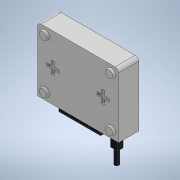
# Autodesk Inventor part: RB941-2nD
Saved by Autodesk Inventor 2022 (Build 260153000, 153)
## iProperties
Created: 2017-05-26
Part Number: RB941-2nD
Material: Ogólne
Document SubType Name: Modeling
Designer: SewerLight
Density: 1 g/cm^3
Appearance: Domyślne
Author: SewerLight
Autodesk Inventor part; units mm, degrees
ref_plane "XZ Plane" through (0, 0, 0) normal (0, 1, 0) x (-1, 0, 0)
sketch "Szkic1" plane through (0, 0, 0) normal (0, 1, 0) x (-1, 0, 0)
  line L0 (56.5, -44.5) -> (-56.5, -44.5)
  line L1 (-56.5, -44.5) -> (-56.5, 44.5)
  line L2 (-56.5, 44.5) -> (56.5, 44.5)
  line L3 (56.5, 44.5) -> (56.5, -44.5)
  line L4 (56.5, -44.5) -> (-56.5, 44.5) construction
  line L5 (-56.5, -44.5) -> (56.5, 44.5) construction
  point P0 (0, 0)
  dimension "d0" = 113
  dimension "d1" = 89
  constraints: 12 end point, 2 midpoint, 2 parallel, 1 horizontal, 1 perpendicular
  measures "d0" distance of L1.end L2.end
  measures "d1" distance of L0.end L1.end
extrude "Wyciągnięcie proste1" add sketch "Szkic1" along normal blind 28
sketch "Szkic2" plane through (0, 28, 0) normal (0, 1, 0) x (1, 0, 0)
  line L0 (56.5, 44.5) -> (56.5, -44.5) projected
  line L1 (56.5, -44.5) -> (-56.5, -44.5) projected
  line L2 (-56.5, -44.5) -> (-56.5, 44.5) projected
  line L3 (-56.5, 44.5) -> (56.5, 44.5) projected
  line L4 (-56.5, 44.5) -> (56.5, 44.5) construction
  line L5 (56.5, 44.5) -> (56.5, -44.5) construction
  line L6 (56.5, -44.5) -> (-56.5, -44.5) construction
  line L7 (-56.5, -44.5) -> (-56.5, 44.5) construction
  line L8 (-25.5673, 3.2324) -> (-27.2934, 3.2324)
  line L9 (-27.2934, 3.2324) -> (-30.4538, 7.2113)
  line L10 (-30.4538, 7.2113) -> (-31.9773, 7.2113)
  line L11 (-31.9773, 7.2113) -> (-31.9773, 3.2324)
  line L12 (-31.9773, 3.2324) -> (-33.3063, 3.2324)
  line L13 (-33.3063, 3.2324) -> (-33.3063, 13.2324)
  line L14 (-33.3063, 13.2324) -> (-30.7293, 13.2324)
  spline S0 degree 2 poles (-30.7293, 13.2324) (-29.8703, 13.2324) (-28.7115, 13.046) (-28.1848, 12.7056) knots 0 0 0 1 2 2 2
  spline S1 degree 2 poles (-28.1848, 12.7056) (-27.658, 12.3653) (-27.0502, 11.3037) (-27.0502, 10.5176) knots 0 0 0 1 2 2 2
  spline S2 degree 2 poles (-27.0502, 10.5176) (-27.0502, 9.4236) (-28.1686, 7.9406) (-29.1248, 7.5841) knots 0 0 0 1 2 2 2
  line L15 (-29.1248, 7.5841) -> (-25.5673, 3.2324)
  spline S3 degree 2 poles (-28.436, 10.4123) (-28.436, 10.8499) (-28.7439, 11.5225) (-29.0681, 11.7413) knots 0 0 0 1 2 2 2
  spline S4 degree 2 poles (-29.0681, 11.7413) (-29.3517, 11.9277) (-30.1053, 12.0816) (-30.6564, 12.0816) knots 0 0 0 1 2 2 2
  line L16 (-30.6564, 12.0816) -> (-31.9773, 12.0816)
  line L17 (-31.9773, 12.0816) -> (-31.9773, 8.3215)
  line L18 (-31.9773, 8.3215) -> (-30.8104, 8.3215)
  spline S5 degree 2 poles (-30.8104, 8.3215) (-30.235, 8.3215) (-29.3193, 8.5241) (-29.0032, 8.8401) knots 0 0 0 1 2 2 2
  spline S6 degree 2 poles (-29.0032, 8.8401) (-28.7115, 9.1157) (-28.436, 9.8936) (-28.436, 10.4123) knots 0 0 0 1 2 2 2
  spline S7 degree 2 poles (-17.9903, 6.3037) (-17.9903, 5.5581) (-18.5575, 4.4155) (-19.0276, 4.0427) knots 0 0 0 1 2 2 2
  spline S8 degree 2 poles (-19.0276, 4.0427) (-19.5948, 3.6051) (-20.8833, 3.2324) (-21.9044, 3.2324) knots 0 0 0 1 2 2 2
  line L19 (-21.9044, 3.2324) -> (-24.7731, 3.2324)
  line L20 (-24.7731, 3.2324) -> (-24.7731, 13.2324)
  line L21 (-24.7731, 13.2324) -> (-22.1232, 13.2324)
  spline S9 degree 2 poles (-22.1232, 13.2324) (-21.0535, 13.2324) (-19.9838, 13.0946) (-19.4976, 12.8272) knots 0 0 0 1 2 2 2
  spline S10 degree 2 poles (-19.4976, 12.8272) (-18.9546, 12.5436) (-18.4603, 11.6116) (-18.4603, 10.9795) knots 0 0 0 1 2 2 2
  spline S11 degree 2 poles (-18.4603, 10.9795) (-18.4603, 10.2745) (-19.2058, 9.1562) (-19.8622, 8.8401) knots 0 0 0 1 2 2 2
  line L22 (-19.8622, 8.8401) -> (-19.8622, 8.7915)
  spline S12 degree 2 poles (-19.8622, 8.7915) (-18.9708, 8.5484) (-17.9903, 7.2599) (-17.9903, 6.3037) knots 0 0 0 1 2 2 2
  spline S13 degree 2 poles (-19.376, 6.247) (-19.376, 6.8142) (-19.7002, 7.5436) (-20.1864, 7.8029) knots 0 0 0 1 2 2 2
  spline S14 degree 2 poles (-20.1864, 7.8029) (-20.5024, 7.9649) (-21.248, 8.0622) (-21.9368, 8.0622) knots 0 0 0 1 2 2 2
  line L23 (-21.9368, 8.0622) -> (-23.4441, 8.0622)
  line L24 (-23.4441, 8.0622) -> (-23.4441, 4.3669)
  line L25 (-23.4441, 4.3669) -> (-22.3663, 4.3669)
  spline S15 degree 2 poles (-22.3663, 4.3669) (-21.4911, 4.3669) (-20.4862, 4.529) (-20.0972, 4.7883) knots 0 0 0 1 2 2 2
  spline S16 degree 2 poles (-20.0972, 4.7883) (-19.7245, 5.0557) (-19.376, 5.7202) (-19.376, 6.247) knots 0 0 0 1 2 2 2
  spline S17 degree 2 poles (-19.846, 10.7931) (-19.846, 11.1497) (-20.0891, 11.6846) (-20.3566, 11.8385) knots 0 0 0 1 2 2 2
  spline S18 degree 2 poles (-20.3566, 11.8385) (-20.6807, 12.0168) (-21.4668, 12.0978) (-22.1718, 12.0978) knots 0 0 0 1 2 2 2
  line L26 (-22.1718, 12.0978) -> (-23.4441, 12.0978)
  line L27 (-23.4441, 12.0978) -> (-23.4441, 9.1724)
  line L28 (-23.4441, 9.1724) -> (-21.9368, 9.1724)
  spline S19 degree 2 poles (-21.9368, 9.1724) (-21.3128, 9.1724) (-20.7212, 9.3021) (-20.4052, 9.5047) knots 0 0 0 1 2 2 2
  spline S20 degree 2 poles (-20.4052, 9.5047) (-20.0972, 9.6991) (-19.846, 10.3231) (-19.846, 10.7931) knots 0 0 0 1 2 2 2
  spline S21 degree 2 poles (-17.2285, 9.9828) (-17.2285, 10.7526) (-16.7261, 12.033) (-16.2885, 12.4949) knots 0 0 0 1 2 2 2
  spline S22 degree 2 poles (-16.2885, 12.4949) (-15.8752, 12.9406) (-14.6677, 13.435) (-14.0519, 13.435) knots 0 0 0 1 2 2 2
  spline S23 degree 2 poles (-14.0519, 13.435) (-13.363, 13.435) (-12.2447, 12.973) (-11.8314, 12.5354) knots 0 0 0 1 2 2 2
  spline S24 degree 2 poles (-11.8314, 12.5354) (-11.3128, 11.9844) (-10.7455, 10.2016) (-10.7455, 8.832) knots 0 0 0 1 2 2 2
  spline S25 degree 2 poles (-10.7455, 8.832) (-10.7455, 7.5922) (-11.3047, 5.3718) (-11.8476, 4.6343) knots 0 0 0 1 2 2 2
  spline S26 degree 2 poles (-11.8476, 4.6343) (-12.423, 3.8564) (-14.0438, 3.0379) (-15.2269, 3.0379) knots 0 0 0 1 2 2 2
  spline S27 degree 2 poles (-15.2269, 3.0379) (-15.4943, 3.0379) (-16.1021, 3.0946) (-16.3614, 3.1756) knots 0 0 0 1 2 2 2
  line L29 (-16.3614, 3.1756) -> (-16.3614, 4.4641)
  line L30 (-16.3614, 4.4641) -> (-16.2966, 4.4641)
  spline S28 degree 2 poles (-16.2966, 4.4641) (-16.1264, 4.3669) (-15.4133, 4.1967) (-15.0486, 4.1967) knots 0 0 0 1 2 2 2
  spline S29 degree 2 poles (-15.0486, 4.1967) (-13.7358, 4.1967) (-12.2366, 5.9309) (-12.1313, 7.5354) knots 0 0 0 1 2 2 2
  spline S30 degree 2 poles (-12.1313, 7.5354) (-12.6661, 7.1708) (-13.6386, 6.8385) (-14.2139, 6.8385) knots 0 0 0 1 2 2 2
  spline S31 degree 2 poles (-14.2139, 6.8385) (-14.765, 6.8385) (-15.6807, 7.0816) (-16.1426, 7.4301) knots 0 0 0 1 2 2 2
  spline S32 degree 2 poles (-16.1426, 7.4301) (-16.6775, 7.8434) (-17.2285, 9.0995) (-17.2285, 9.9828) knots 0 0 0 1 2 2 2
  spline S33 degree 2 poles (-12.0989, 9.1319) (-12.0989, 10.1448) (-12.4716, 11.4252) (-12.8039, 11.7737) knots 0 0 0 1 2 2 2
  spline S34 degree 2 poles (-12.8039, 11.7737) (-13.0956, 12.0978) (-13.7034, 12.341) (-14.06, 12.341) knots 0 0 0 1 2 2 2
  spline S35 degree 2 poles (-14.06, 12.341) (-14.8865, 12.341) (-15.8671, 11.1578) (-15.8671, 10.0395) knots 0 0 0 1 2 2 2
  spline S36 degree 2 poles (-15.8671, 10.0395) (-15.8671, 9.4074) (-15.5429, 8.5889) (-15.1864, 8.2972) knots 0 0 0 1 2 2 2
  spline S37 degree 2 poles (-15.1864, 8.2972) (-14.9271, 8.0865) (-14.2869, 7.9487) (-13.9141, 7.9487) knots 0 0 0 1 2 2 2
  spline S38 degree 2 poles (-13.9141, 7.9487) (-13.4846, 7.9487) (-12.4959, 8.2486) (-12.1232, 8.4998) knots 0 0 0 1 2 2 2
  spline S39 degree 2 poles (-12.1232, 8.4998) (-12.1151, 8.597) (-12.0989, 8.9293) (-12.0989, 9.1319) knots 0 0 0 1 2 2 2
  line L31 (-3.0146, 6.6683) -> (-4.2058, 6.6683)
  line L32 (-4.2058, 6.6683) -> (-4.2058, 3.2324)
  line L33 (-4.2058, 3.2324) -> (-5.4943, 3.2324)
  line L34 (-5.4943, 3.2324) -> (-5.4943, 6.6683)
  line L35 (-5.4943, 6.6683) -> (-9.9109, 6.6683)
  line L36 (-9.9109, 6.6683) -> (-9.9109, 8.0784)
  line L37 (-9.9109, 8.0784) -> (-5.4376, 13.2324)
  line L38 (-5.4376, 13.2324) -> (-4.2058, 13.2324)
  line L39 (-4.2058, 13.2324) -> (-4.2058, 7.7461)
  line L40 (-4.2058, 7.7461) -> (-3.0146, 7.7461)
  line L41 (-3.0146, 7.7461) -> (-3.0146, 6.6683)
  line L42 (-5.4943, 7.7461) -> (-5.4943, 11.6521)
  line L43 (-5.4943, 11.6521) -> (-8.8574, 7.7461)
  line L44 (-8.8574, 7.7461) -> (-5.4943, 7.7461)
  line L45 (3.7196, 3.2324) -> (-1.1588, 3.2324)
  line L46 (-1.1588, 3.2324) -> (-1.1588, 4.2534)
  line L47 (-1.1588, 4.2534) -> (0.6564, 4.2534)
  line L48 (0.6564, 4.2534) -> (0.6564, 10.9552)
  line L49 (0.6564, 10.9552) -> (-1.1588, 10.9552)
  line L50 (-1.1588, 10.9552) -> (-1.1588, 11.8709)
  spline S40 degree 2 poles (-1.1588, 11.8709) (-0.1297, 11.8709) (0.8428, 12.4544) (0.9076, 13.2648) knots 0 0 0 1 2 2 2
  line L51 (0.9076, 13.2648) -> (1.9449, 13.2648)
  line L52 (1.9449, 13.2648) -> (1.9449, 4.2534)
  line L53 (1.9449, 4.2534) -> (3.7196, 4.2534)
  line L54 (3.7196, 4.2534) -> (3.7196, 3.2324)
  line L55 (9.222, 7.0006) -> (5.4376, 7.0006)
  line L56 (5.4376, 7.0006) -> (5.4376, 8.2162)
  line L57 (5.4376, 8.2162) -> (9.222, 8.2162)
  line L58 (9.222, 8.2162) -> (9.222, 7.0006)
  line L59 (16.718, 3.2324) -> (10.5511, 3.2324)
  line L60 (10.5511, 3.2324) -> (10.5511, 4.6505)
  spline S41 degree 2 poles (10.5511, 4.6505) (11.2156, 5.2745) (12.3987, 6.4333) (12.966, 7.0573) knots 0 0 0 1 2 2 2
  spline S42 degree 2 poles (12.966, 7.0573) (14.1086, 8.3134) (14.9433, 9.8207) (14.9433, 10.623) knots 0 0 0 1 2 2 2
  spline S43 degree 2 poles (14.9433, 10.623) (14.9433, 11.0444) (14.684, 11.6765) (14.4489, 11.879) knots 0 0 0 1 2 2 2
  spline S44 degree 2 poles (14.4489, 11.879) (14.2139, 12.0816) (13.5981, 12.2842) (13.2253, 12.2842) knots 0 0 0 1 2 2 2
  spline S45 degree 2 poles (13.2253, 12.2842) (12.8687, 12.2842) (12.1394, 12.106) (11.8071, 11.9682) knots 0 0 0 1 2 2 2
  spline S46 degree 2 poles (11.8071, 11.9682) (11.5235, 11.8547) (10.9968, 11.5306) (10.8347, 11.4171) knots 0 0 0 1 2 2 2
  line L61 (10.8347, 11.4171) -> (10.7618, 11.4171)
  line L62 (10.7618, 11.4171) -> (10.7618, 12.8434)
  spline S47 degree 2 poles (10.7618, 12.8434) (11.175, 13.046) (12.658, 13.4431) (13.3225, 13.4431) knots 0 0 0 1 2 2 2
  spline S48 degree 2 poles (13.3225, 13.4431) (14.7245, 13.4431) (16.3047, 11.9601) (16.3047, 10.6959) knots 0 0 0 1 2 2 2
  spline S49 degree 2 poles (16.3047, 10.6959) (16.3047, 10.1043) (16.0292, 9.1157) (15.7861, 8.6943) knots 0 0 0 1 2 2 2
  spline S50 degree 2 poles (15.7861, 8.6943) (15.543, 8.2567) (14.8379, 7.3977) (14.4489, 6.9844) knots 0 0 0 1 2 2 2
  spline S51 degree 2 poles (14.4489, 6.9844) (13.8169, 6.2956) (12.269, 4.8207) (11.8071, 4.3912) knots 0 0 0 1 2 2 2
  line L63 (11.8071, 4.3912) -> (16.718, 4.3912)
  line L64 (16.718, 4.3912) -> (16.718, 3.2324)
  line L65 (24.1329, 3.2324) -> (22.8687, 3.2324)
  line L66 (22.8687, 3.2324) -> (22.8687, 7.5111)
  spline S52 degree 2 poles (22.8687, 7.5111) (22.8687, 8.0298) (22.7715, 8.9212) (22.6256, 9.1886) knots 0 0 0 1 2 2 2
  spline S53 degree 2 poles (22.6256, 9.1886) (22.4716, 9.4722) (21.9206, 9.7478) (21.4506, 9.7478) knots 0 0 0 1 2 2 2
  spline S54 degree 2 poles (21.4506, 9.7478) (20.9806, 9.7478) (19.9838, 9.2453) (19.5057, 8.8401) knots 0 0 0 1 2 2 2
  line L67 (19.5057, 8.8401) -> (19.5057, 3.2324)
  line L68 (19.5057, 3.2324) -> (18.2415, 3.2324)
  line L69 (18.2415, 3.2324) -> (18.2415, 10.7364)
  line L70 (18.2415, 10.7364) -> (19.5057, 10.7364)
  line L71 (19.5057, 10.7364) -> (19.5057, 9.9017)
  spline S55 degree 2 poles (19.5057, 9.9017) (20.0729, 10.4123) (21.1669, 10.9471) (21.7828, 10.9471) knots 0 0 0 1 2 2 2
  spline S56 degree 2 poles (21.7828, 10.9471) (22.8849, 10.9471) (24.1329, 9.4884) (24.1329, 8.1027) knots 0 0 0 1 2 2 2
  line L72 (24.1329, 8.1027) -> (24.1329, 3.2324)
  spline S57 degree 2 poles (33.8898, 8.2243) (33.8898, 6.8547) (32.7796, 4.6505) (31.8477, 4.0346) knots 0 0 0 1 2 2 2
  spline S58 degree 2 poles (31.8477, 4.0346) (31.0859, 3.5565) (29.5219, 3.2324) (28.3063, 3.2324) knots 0 0 0 1 2 2 2
  line L73 (28.3063, 3.2324) -> (26.0049, 3.2324)
  line L74 (26.0049, 3.2324) -> (26.0049, 13.2324)
  line L75 (26.0049, 13.2324) -> (28.282, 13.2324)
  spline S59 degree 2 poles (28.282, 13.2324) (29.6921, 13.2324) (31.2966, 12.811) (31.8639, 12.4382) knots 0 0 0 1 2 2 2
  spline S60 degree 2 poles (31.8639, 12.4382) (32.8282, 11.798) (33.8898, 9.6829) (33.8898, 8.2243) knots 0 0 0 1 2 2 2
  spline S61 degree 2 poles (32.5041, 8.2405) (32.5041, 9.3912) (31.7423, 11.0201) (30.9887, 11.482) knots 0 0 0 1 2 2 2
  spline S62 degree 2 poles (30.9887, 11.482) (30.4538, 11.798) (29.2464, 12.0816) (28.3468, 12.0816) knots 0 0 0 1 2 2 2
  line L76 (28.3468, 12.0816) -> (27.3339, 12.0816)
  line L77 (27.3339, 12.0816) -> (27.3339, 4.3831)
  line L78 (27.3339, 4.3831) -> (28.3468, 4.3831)
  spline S63 degree 2 poles (28.3468, 4.3831) (29.2301, 4.3831) (30.5673, 4.6667) (31.1102, 5.0476) knots 0 0 0 1 2 2 2
  spline S64 degree 2 poles (31.1102, 5.0476) (31.8071, 5.5176) (32.5041, 7.0735) (32.5041, 8.2405) knots 0 0 0 1 2 2 2
  line L79 (-15.9319, -13.2324) -> (-17.2609, -13.2324)
  line L80 (-17.2609, -13.2324) -> (-17.2609, -4.6181)
  line L81 (-17.2609, -4.6181) -> (-19.8703, -10.4771)
  line L82 (-19.8703, -10.4771) -> (-20.6807, -10.4771)
  line L83 (-20.6807, -10.4771) -> (-23.2658, -4.6181)
  line L84 (-23.2658, -4.6181) -> (-23.2658, -13.2324)
  line L85 (-23.2658, -13.2324) -> (-24.5057, -13.2324)
  line L86 (-24.5057, -13.2324) -> (-24.5057, -3.2324)
  line L87 (-24.5057, -3.2324) -> (-22.6904, -3.2324)
  line L88 (-22.6904, -3.2324) -> (-20.1945, -8.7996)
  line L89 (-20.1945, -8.7996) -> (-17.7796, -3.2324)
  line L90 (-17.7796, -3.2324) -> (-15.9319, -3.2324)
  line L91 (-15.9319, -3.2324) -> (-15.9319, -13.2324)
  line L92 (-12.7147, -13.2324) -> (-13.9789, -13.2324)
  line L93 (-13.9789, -13.2324) -> (-13.9789, -5.7283)
  line L94 (-13.9789, -5.7283) -> (-12.7147, -5.7283)
  line L95 (-12.7147, -5.7283) -> (-12.7147, -13.2324)
  line L96 (-12.6256, -4.4803) -> (-14.06, -4.4803)
  line L97 (-14.06, -4.4803) -> (-14.06, -3.1675)
  line L98 (-14.06, -3.1675) -> (-12.6256, -3.1675)
  line L99 (-12.6256, -3.1675) -> (-12.6256, -4.4803)
  line L100 (-4.6434, -13.2324) -> (-6.3047, -13.2324)
  line L101 (-6.3047, -13.2324) -> (-9.0924, -9.61)
  line L102 (-9.0924, -9.61) -> (-9.5948, -10.0962)
  line L103 (-9.5948, -10.0962) -> (-9.5948, -13.2324)
  line L104 (-9.5948, -13.2324) -> (-10.859, -13.2324)
  line L105 (-10.859, -13.2324) -> (-10.859, -2.7867)
  line L106 (-10.859, -2.7867) -> (-9.5948, -2.7867)
  line L107 (-9.5948, -2.7867) -> (-9.5948, -8.8969)
  line L108 (-9.5948, -8.8969) -> (-6.6288, -5.7283)
  line L109 (-6.6288, -5.7283) -> (-5.0567, -5.7283)
  line L110 (-5.0567, -5.7283) -> (-8.1361, -8.8645)
  line L111 (-8.1361, -8.8645) -> (-4.6434, -13.2324)
  line L112 (-0.0324, -7.0816) -> (-0.0972, -7.0816)
  spline S65 degree 2 poles (-0.0972, -7.0816) (-0.2431, -7.0411) (-0.5592, -7.0249) (-0.778, -7.0249) knots 0 0 0 1 2 2 2
  spline S66 degree 2 poles (-0.778, -7.0249) (-1.2885, -7.0249) (-2.2934, -7.4706) (-2.7472, -7.9082) knots 0 0 0 1 2 2 2
  line L113 (-2.7472, -7.9082) -> (-2.7472, -13.2324)
  line L114 (-2.7472, -13.2324) -> (-4.0113, -13.2324)
  line L115 (-4.0113, -13.2324) -> (-4.0113, -5.7283)
  line L116 (-4.0113, -5.7283) -> (-2.7472, -5.7283)
  line L117 (-2.7472, -5.7283) -> (-2.7472, -6.8466)
  spline S67 degree 2 poles (-2.7472, -6.8466) (-2.0583, -6.2307) (-1.0292, -5.7283) (-0.543, -5.7283) knots 0 0 0 1 2 2 2
  spline S68 degree 2 poles (-0.543, -5.7283) (-0.3485, -5.7283) (-0.154, -5.7445) (-0.0324, -5.7688) knots 0 0 0 1 2 2 2
  line L118 (-0.0324, -5.7688) -> (-0.0324, -7.0816)
  spline S69 degree 2 poles (7.1151, -9.4803) (7.1151, -11.3766) (5.2917, -13.4431) (3.7682, -13.4431) knots 0 0 0 1 2 2 2
  spline S70 degree 2 poles (3.7682, -13.4431) (2.2042, -13.4431) (0.4133, -11.3118) (0.4133, -9.4803) knots 0 0 0 1 2 2 2
  spline S71 degree 2 poles (0.4133, -9.4803) (0.4133, -7.6003) (2.2609, -5.5176) (3.7682, -5.5176) knots 0 0 0 1 2 2 2
  spline S72 degree 2 poles (3.7682, -5.5176) (5.2917, -5.5176) (7.1151, -7.5922) (7.1151, -9.4803) knots 0 0 0 1 2 2 2
  spline S73 degree 2 poles (5.8104, -9.4803) (5.8104, -8.0217) (4.7488, -6.6035) (3.7682, -6.6035) knots 0 0 0 1 2 2 2
  spline S74 degree 2 poles (3.7682, -6.6035) (2.7877, -6.6035) (1.718, -8.0217) (1.718, -9.4803) knots 0 0 0 1 2 2 2
  spline S75 degree 2 poles (1.718, -9.4803) (1.718, -10.8985) (2.7877, -12.3572) (3.7682, -12.3572) knots 0 0 0 1 2 2 2
  spline S76 degree 2 poles (3.7682, -12.3572) (4.7407, -12.3572) (5.8104, -10.9228) (5.8104, -9.4803) knots 0 0 0 1 2 2 2
  line L119 (10.8428, -13.2324) -> (10.8428, -4.4155)
  line L120 (10.8428, -4.4155) -> (7.4878, -4.4155)
  line L121 (7.4878, -4.4155) -> (7.4878, -3.2324)
  line L122 (7.4878, -3.2324) -> (15.5267, -3.2324)
  line L123 (15.5267, -3.2324) -> (15.5267, -4.4155)
  line L124 (15.5267, -4.4155) -> (12.1718, -4.4155)
  line L125 (12.1718, -4.4155) -> (12.1718, -13.2324)
  line L126 (12.1718, -13.2324) -> (10.8428, -13.2324)
  line L127 (17.731, -13.2324) -> (16.4668, -13.2324)
  line L128 (16.4668, -13.2324) -> (16.4668, -5.7283)
  line L129 (16.4668, -5.7283) -> (17.731, -5.7283)
  line L130 (17.731, -5.7283) -> (17.731, -13.2324)
  line L131 (17.8201, -4.4803) -> (16.3857, -4.4803)
  line L132 (16.3857, -4.4803) -> (16.3857, -3.1675)
  line L133 (16.3857, -3.1675) -> (17.8201, -3.1675)
  line L134 (17.8201, -3.1675) -> (17.8201, -4.4803)
  line L135 (25.8023, -13.2324) -> (24.141, -13.2324)
  line L136 (24.141, -13.2324) -> (21.3533, -9.61)
  line L137 (21.3533, -9.61) -> (20.8509, -10.0962)
  line L138 (20.8509, -10.0962) -> (20.8509, -13.2324)
  line L139 (20.8509, -13.2324) -> (19.5867, -13.2324)
  line L140 (19.5867, -13.2324) -> (19.5867, -2.7867)
  line L141 (19.5867, -2.7867) -> (20.8509, -2.7867)
  line L142 (20.8509, -2.7867) -> (20.8509, -8.8969)
  line L143 (20.8509, -8.8969) -> (23.8169, -5.7283)
  line L144 (23.8169, -5.7283) -> (25.389, -5.7283)
  line L145 (25.389, -5.7283) -> (22.3096, -8.8645)
  line L146 (22.3096, -8.8645) -> (25.8023, -13.2324)
  point P0 (0, 0)
  constraints: 2 coincident, 2 other
emboss "Wypukłość1" sketch "Szkic2" operation add depth 0.1 direction (0, -1, 0) contours L8 L9 L10 L11 L12 L13 L14 S0 S1 S2 L15 | S7 S8 L19 L20 L21 S9 S10 S11 L22 S12 | S21 S22 S23 S24 S25 S26 S27 L29 L30 S28 S29 S30 S31 S32 | L31 L32 L33 L34 L35 L36 L37 L38 L39 L40 L41 | L45 L46 L47 L48 L49 L50 S40 L51 L52 L53 L54 | L55 L56 L57 L58 | L59 L60 S41 S42 S43 S44 S45 S46 L61 L62 S47 S48 S49 S50 S51 L63 L64 | L65 L66 S52 S53 S54 L67 L68 L69 L70 L71 S55 S56 L72 | S57 S58 L73 L74 L75 S59 S60 | L79 L80 L81 L82 L83 L84 L85 L86 L87 L88 L89 L90 L91 | L92 L93 L94 L95 | L96 L97 L98 L99 | L100 L101 L102 L103 L104 L105 L106 L107 L108 L109 L110 L111 | L112 S65 S66 L113 L114 L115 L116 L117 S67 S68 L118 | S69 S70 S71 S72 | L119 L120 L121 L122 L123 L124 L125 L126 | L127 L128 L129 L130 | L131 L132 L133 L134 | L135 L136 L137 L138 L139 L140 L141 L142 L143 L144 L145 L146
sketch "Szkic5" plane through (0, 0, 0) normal (0, -1, 0) x (1, 0, 0)
  circle A0 centre (-46, 34.5) radius 6
  point P0 (0, 0)
  dimension "d14" = 12
  dimension "d15" = 46
  dimension "d16" = 34.5
  constraints: 1 centre point
  measures "d14" diameter of A0
  measures "d15" horizontal distance of point (0, 0) A0.centre
  measures "d16" vertical distance of point (0, 0) A0.centre
extrude "Wyciągnięcie proste4" add sketch "Szkic5" along normal blind 2.9
draft "Pochylenie ściany1" angle 15 pull direction (0, -1, 0) faces at (-40.0195, -1.9333, 34.0172) fixed edges at (-52, 0, 34.5)
mirror "Odbij1" about plane through (0, 0, 0) normal (0, 0, 1) of "Wyciągnięcie proste4", "Pochylenie ściany1"
sketch "Szkic3" plane through (0, 0, 0) normal (0, -1, 0) x (1, 0, 0)
  line L0 (-37.05, -2.05) -> (-43.65, -2.05)
  line L1 (-43.65, -2.05) -> (-43.65, 2.05)
  line L2 (-43.65, 2.05) -> (-37.05, 2.05)
  line L3 (-37.05, 2.05) -> (-37.05, 8.65)
  line L4 (-37.05, 8.65) -> (-32.95, 8.65)
  line L5 (-32.95, 8.65) -> (-32.95, 2.05)
  line L6 (-32.95, 2.05) -> (-26.35, 2.05)
  line L7 (-26.35, 2.05) -> (-26.35, -2.05)
  line L8 (-26.35, -2.05) -> (-32.95, -2.05)
  line L9 (-32.95, -2.05) -> (-32.95, -8.65)
  line L10 (-32.95, -8.65) -> (-37.05, -8.65)
  line L11 (-37.05, -8.65) -> (-37.05, -2.05)
  line L12 (-26.35, 0) -> (0, 0) construction
  dimension "d6" = 26.35
  dimension "d7" = 4.1
  dimension "d8" = 17.3
  constraints: 26 end point, 13 perpendicular, 5 point on line, 2 horizontal, 1 collinear, 1 midpoint
  measures "d6" distance of L12.start L12.end
  measures "d7" distance of L9.end L10.end
  measures "d8" distance between parallel lines of L7 L1
extrude "Wyciągnięcie proste2" cut sketch "Szkic3" against normal blind 3.6
ref_plane "Płaszczyzna konstrukcyjna1" through (0, 1, 0) normal (0, -1, 0) x (1, 0, 0)
sketch "Szkic4" plane through (0, 1, 0) normal (0, -1, 0) x (1, 0, 0)
  line L0 (-37.05, 2.05) -> (-37.05, 8.65) construction
  line L1 (-26.35, -2.05) -> (-32.95, -2.05) construction
  line L2 (-37.05, 2.05) -> (-32.95, -2.05) construction
  circle A0 centre (-35, 0) radius 8.65
  line L3 (-26.35, 2.05) -> (-26.35, -2.05) projected
  point P0 (0, 0)
  constraints: 2 end point, 1 centre point, 1 midpoint, 1 tangent
extrude "Wyciągnięcie proste3" cut sketch "Szkic4" against normal up to surface (2.6 mm away)
mirror "Odbij2" about plane through (0, 0, 0) normal (1, 0, 0) of "Wyciągnięcie proste4", "Pochylenie ściany1", "Odbij1", "Wyciągnięcie proste2", "Wyciągnięcie proste3"
fillet "Zaokrąglenie1" radius 5 2 edges at (-56.5, 14, 44.5) (56.5, 14, 44.5)
sketch "Szkic8" plane through (56.5, 0, -44.5) normal (0, 0, -1) x (-1, 0, 0)
  line L0 (39, 21) -> (52.3, 21)
  line L1 (52.3, 21) -> (52.3, 12)
  line L2 (52.3, 12) -> (39, 12)
  line L3 (39, 12) -> (39, 21)
  line L4 (0, 28) -> (113, 28) projected
  line L5 (0, 0) -> (0, 28) projected
  point P0 (56.5, 0)
  dimension "d30" = 13.3
  dimension "d31" = 9
  dimension "d32" = 7
  dimension "d33" = 39
  constraints: 8 end point, 2 parallel, 1 horizontal, 1 perpendicular
  measures "d30" distance of L1.end L2.end
  measures "d31" distance of L0.end L1.end
  measures "d32" distance between parallel lines of L0 L4
  measures "d33" distance between parallel lines of L5 L3
ref_plane "Płaszczyzna konstrukcyjna2" through (10.85, 0, 0) normal (1, 0, 0) x (0, 1, 0)
sketch "Szkic9" plane through (10.85, 0, 0) normal (1, 0, 0) x (0, 1, 0)
  line L0 (21, -44.5) -> (12, -44.5) projected
  line L1 (16.5, -44.5) -> (16.5, -58.2)
  line L2 (16.5, -58.2) -> (36, -58.2)
  point P0 (0, 0)
  dimension "d35" = 13.7
  dimension "d36" = 19.5
  constraints: 4 end point, 1 horizontal, 1 midpoint, 1 vertical
  measures "d35" distance of L1.start L1.end
  measures "d36" distance of L1.end L2.end
sweep "Przeciągnięcie1" add profiles "Szkic8" path "Szkic9" path curves L1 L2
sketch "Szkic6" plane through (56.5, 0, -44.5) normal (0, 0, -1) x (-1, 0, 0)
  line L0 (5.5, 11.8) -> (15.5, 11.8)
  line L1 (15.5, 11.8) -> (15.5, 4)
  line L2 (15.5, 4) -> (5.5, 4)
  line L3 (5.5, 4) -> (5.5, 11.8)
  line L4 (0, 28) -> (0, 0)
  line L5 (113, 0) -> (0.4162, 0)
  line L6 (113, 0) -> (0, 0) projected
  line L7 (0, 0) -> (0, 28) projected
  point P0 (51.5, 0)
  dimension "d21" = 10
  dimension "d22" = 7.8
  dimension "d23" = 5.5
  dimension "d24" = 4
  constraints: 12 end point, 2 collinear, 2 parallel, 1 horizontal, 1 perpendicular
  measures "d21" distance of L1.end L2.end
  measures "d22" distance of L0.end L1.end
  measures "d23" distance between parallel lines of L3 L4
  measures "d24" distance between parallel lines of L5 L2
extrude "Wyciągnięcie proste5" add sketch "Szkic6" along normal blind 15
sketch "Szkic7" plane through (56.5, 0, -59.5) normal (0, 0, -1) x (-1, 0, 0)
  line L0 (15.5, 11.8) -> (5.5, 11.8) projected
  line L1 (5.5, 11.8) -> (5.5, 4) projected
  line L2 (5.5, 4) -> (15.5, 4) projected
  line L3 (15.5, 4) -> (15.5, 11.8) projected
  line L4 (5.5, 4) -> (15.5, 11.8) construction
  circle A0 centre (10.5, 7.9) radius 3.15
  point P0 (56.5, 0)
  dimension "d27" = 6.3
  constraints: 2 end point, 1 centre point, 1 midpoint
  measures "d27" diameter of A0
extrude "Wyciągnięcie proste6" add sketch "Szkic7" along normal blind 20 contours A0
fillet "Zaokrąglenie2" radius 3 2 edges at (10.85, 12, -62.7) (10.85, 21, -53.7)
chamfer "Faza1" distance 3 distance2 10 1 edges at (17.5, 36, -58.2) measured on face at (17, 36, -58.2)
chamfer "Faza2" distance 3 distance2 10 1 edges at (4.2, 36, -58.2) measured on face at (4.7, 36, -58.2)
pattern_linear "Szyk prostokątny1" count 4 spacing 14.4 along (-1, 0, 0) of "Przeciągnięcie1", "Faza2", "Faza1", "Zaokrąglenie2"
